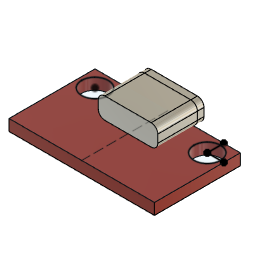
usbc v10 (Autodesk Fusion 360 design; units mm, degrees)
Autodesk Fusion 360 part; units mm, degrees
note: some values were not read from the file. Set by a fixed rule: which sketch regions a step uses.
sketch "Sketch1" plane through (0, 0, 0) normal (0, 0, 1) x (1, 0, 0) in component "board"
  line L0 (11, -6.5) -> (-11, -6.5)
  line L1 (-11, -6.5) -> (-11, 6.5)
  line L2 (-11, 6.5) -> (11, 6.5)
  line L3 (11, 6.5) -> (11, -6.5)
  line L4 (11, -6.5) -> (-11, 6.5) construction
  line L5 (-11, -6.5) -> (11, 6.5) construction
  dimension "d1" = 22
  dimension "d2" = 13
  constraint horizontal L0
  constraint perpendicular L0 L1
  constraint parallel L0 L2
  constraint parallel L1 L3
  constraint coincident L4 origin
  constraint coincident L5 origin
  measures "d1" distance of L0.start L0.end
  measures "d2" distance of L0.start L2.end
extrude "Extrude1" add sketch "Sketch1" along normal blind 1.7 makes body 1 in component "board"
sketch "Sketch1 (2)" plane through (0, 0, 1.7) normal (0, 0, 1) x (-1, 0, 0) in component "port"
  line L0 (-11, -6.5) -> (11, -6.5)
  line L1 (11, -6.5) -> (11, 6.5)
  line L2 (11, 6.5) -> (-11, 6.5)
  line L3 (-11, 6.5) -> (-11, -6.5)
  line L4 (4.5, -7.5) -> (-4.5, -7.5)
  line L5 (-4.5, -7.5) -> (-4.5, -0.5)
  line L6 (-4.5, -0.5) -> (4.5, -0.5)
  line L7 (4.5, -0.5) -> (4.5, -7.5)
  line L8 (11, -6.5) -> (-11, -6.5)
  line L9 (-4.5, -3.3996) -> (-11, -3.3996) construction
  line L10 (4.5, -3.3996) -> (11, -3.3996) construction
  dimension "d12" = 9
  dimension "d13" = 7
  dimension "d20" = 1
  constraint horizontal L4
  constraint vertical L5
  constraint horizontal L6
  constraint vertical L7
  constraint coincident L5 L9.start
  constraint coincident L3 L9.end
  constraint perpendicular L3 L9
  constraint coincident L7 L10.start
  constraint coincident L1 L10.end
  constraint perpendicular L1 L10
  constraint equal L9 L10
  measures "d12" distance of L4.start L4.end
  measures "d13" distance of L4.start L6.end
  measures "d20" distance of L4 L8
extrude "Extrude2" add sketch "Sketch1 (2)" along normal blind 3.2 separate body contours L0 L4 L5 L7 L8 makes body 2 in component "port"
extrude "Extrude1'" add sketch "Sketch1 (2)" along normal blind 3.2 separate body contours L0 L5 L6 L7 L8 makes body 3 in component "port"
fillet "Fillet1" radius 1 8 edges at (4.5, 3.5, 4.9) (4.5, 3.5, 1.7) (-4.5, 3.5, 1.7) (-4.5, 3.5, 4.9) (4.5, 7, 4.9) (4.5, 7, 1.7) (-4.5, 7, 1.7) (-4.5, 7, 4.9) on bodies 2 3 in component "port"
sketch "Sketch1 (3)" plane through (0, 0, 1.7) normal (0, 0, 1) x (-1, 0, 0)
  line L0 (-11, -6.5) -> (11, -6.5)
  line L1 (11, -6.5) -> (11, 6.5)
  line L2 (11, 6.5) -> (-11, 6.5)
  line L3 (-11, 6.5) -> (-11, -6.5)
  circle A0 centre (-8.5, -4) radius 2
  line L4 (-8.5, -4) -> (-8.5, -6.5)
  line L5 (-8.5, -4) -> (-11, -4)
  line L6 (0, -6.5) -> (0, 6.5) construction
  circle A1 centre (8.5, -4) radius 2
  dimension "d24" = 4
  dimension "d25" = 2.5
  dimension "d28" = 2.5
  constraint coincident A0.centre L4.start
  constraint coincident L0 L4.end
  constraint perpendicular L0 L4
  constraint coincident L3 L5.end
  constraint perpendicular L3 L5
  constraint midpoint L0 L6.start
  constraint midpoint L2 L6.end
  constraint symmetric A0 L6 A1
  measures "d24" diameter of A0
  measures "d25" distance of A0.centre L5.end
  measures "d28" distance of A0.centre L4.end
extrude "Extrude4" cut sketch "Sketch1 (3)" against normal up to surface (1.7 mm away) contours A0 L4 L5 | A0 L4 L5 | A1 bodies 1 in component "board"
component "board" placed x (1, 0, 0) y (0, 1, 0) z (0, 0, 1) at (0, 0, 0)
component "port" placed x (1, 0, 0) y (0, 1, 0) z (0, 0, 1) at (0, 0, 0)
